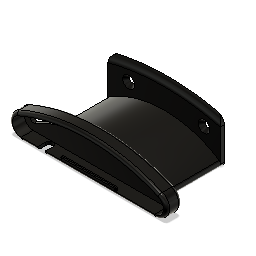
Logitech_g535_Wall_Mount (Autodesk Fusion 360 design; units mm, degrees)
Autodesk Fusion 360 part; units mm, degrees
note: some values were not read from the file. Set by a fixed rule: which face or edge a step refers to.
sketch "Sketch1" plane through (0, 0, 0) normal (0, 0, 1) x (1, 0, 0)
  line L0 (0, 0) -> (101.6, 0)
  line L1 (50.8, 0) -> (50.8, 17.4625)
  arc A0 (101.6, 0) -> (0, 0) centre (50.8, -65.1597) ccw
  dimension "d1" = 101.6
  dimension "d2" = 17.4625
  constraint coincident L0.start A0.end
  constraint horizontal L0
  constraint midpoint L0 L1.start
  constraint perpendicular L0 L1
  constraint coincident L1.end A0
  measures "d1" distance of L0.start L0.end
  measures "d2" distance of L1.start L1.end
extrude "Extrude1" add sketch "Sketch1" along normal blind 50.8 makes body 1
sketch "Sketch2" plane through (0, 0, 50.8) normal (0, 0, 1) x (1, 0, 0)
  arc A0 (101.6, 0) -> (0, 0) centre (50.8, -65.1597) ccw
  line L0 (0, 0) -> (101.6, 0)
  line L1 (0, 0) -> (101.6, 0)
  constraint coincident A0.end L0.start
  constraint coincident A0.start L0.end
copy_body "CopyPasteBodies1" bodies 1 makes body 2
move_body "Move1" bodies 2 to x (1, 0, 0) y (0, 1, 0) z (0, 0, 1) at (0, 40.64, 0)
scale "Scale1" factor 1.453488 about (0, 40.64, 0) bodies 2
sketch "Sketch3" plane through (0, 0, 0) normal (0, 0, -1) x (-1, 0, 0)
  arc A0 (0, 0) -> (-101.6, 0) centre (-50.8, -65.1597) ccw
  line L0 (-101.6, 0) -> (0, 0)
scale "Scale2" factor 1.5 about (0, 40.64, 0) bodies 2
sketch "Sketch4" plane through (0, 0, 0) normal (0, 0, -1) x (-1, 0, 0)
  arc A0 (0, 40.64) -> (-221.5116, 40.64) centre (-110.7558, -101.4232) ccw
  line L0 (-221.5116, 40.64) -> (0, 40.64)
fillet "Fillet1" radius 2.54 2 edges at (0, 0, 25.4) (101.6, 0, 25.4) on bodies 1
copy_body "Body->Comp1" bodies 1 removing the originals makes body 3 in component "Component"
copy_body "Body->Comp2" bodies 2 removing the originals makes body 4 in component "Component'"
scale "Scale1'" factor 0.8 about (221.5116, 40.64, 0) bodies 4 in component "Component'"
fillet "Fillet1'" radius 9.652 2 edges at (44.3023, 40.64, 44.3023) (221.5116, 40.64, 44.3023) on bodies 4 in component "Component'"
extrude "Extrude1'" cut 1 faces at (132.907, 50.7926, 88.6047) along direction (0, 0, -1) blind 76.2 on bodies 4 bodies 4 in component "Component'"
fillet "Fillet2" radius 2.54 8 edges at (132.907, 40.64, 0) (195.9758, 48.3263, 0) (132.907, 71.0978, 0) (69.8382, 48.3263, 0) (132.907, 40.64, 12.4047) (69.8382, 48.3263, 12.4047) (132.907, 71.0978, 12.4047) (195.9758, 48.3263, 12.4047) on bodies 4 in component "Component'"
extrude "Extrude2" cut 1 faces at (132.907, 51.6393, 12.4047) along direction (0, 0, -1) blind 9.652 on bodies 4 bodies 4 in component "Component'"
sketch "Sketch5" plane through (0, 0, 49.0633) normal (0, 0, -1) x (-1, 0, 0)
  line L0 (-104.4191, 2.54) -> (2.8191, 2.54)
  arc A0 (2.8191, 2.54) -> (5.6552, 16.174) centre (2.8191, 9.652) ccw
  arc A1 (5.6552, 16.174) -> (-107.2552, 16.174) centre (-50.8, -113.6506) ccw
  arc A2 (-107.2552, 16.174) -> (-104.4191, 2.54) centre (-104.4191, 9.652) ccw
  arc A3 (1.9271, 8.0079) -> (-103.5271, 8.0079) centre (-50.8, -89.1764) ccw
  arc A4 (1.9271, 8.0079) -> (3.7111, 11.2961) centre (2.8191, 9.652) ccw
  arc A5 (3.7111, 11.2961) -> (-105.3111, 11.2961) centre (-50.8, -89.1764) ccw
  arc A6 (-105.3111, 11.2961) -> (-103.5271, 8.0079) centre (-104.4191, 9.652) ccw
  arc A7 (2.8191, 9.652) -> (-104.4191, 9.652) centre (-50.8, -89.1764) ccw construction
  constraint tangent A3 A4
  constraint tangent A4 A5
  constraint tangent A5 A6
  constraint tangent A3 A6
  constraint coincident A2.centre A6.centre
  constraint coincident A0.centre A4.centre
extrude "Extrude3" cut sketch "Sketch5" against normal blind 23.114 contours A3 A4 A5 A6 sketch seen with x (1, 0, 0) y (0, 1, 0) z (0, 0, 1) at (82.107, 40.64, -49.0633) bodies 4 in component "Component'"
sketch "Sketch6" plane through (0, 0, 0) normal (0, 0, -1) x (-1, 0, 0)
  arc A0 (-94.9342, 4.6873) -> (-93.5774, 0) centre (-93.5774, 2.54) ccw
  line L0 (-93.5774, 0) -> (-8.0226, 0)
  arc A1 (-8.0226, 0) -> (-6.6658, 4.6873) centre (-8.0226, 2.54) ccw
  arc A2 (-6.6658, 4.6873) -> (-94.9342, 4.6873) centre (-50.8, -65.1597) ccw
  line L1 (-93.5774, 0) -> (-8.0226, 0)
  line L2 (-8.0226, 0) -> (-8.0226, 39.4194)
  line L3 (-8.0226, 39.4194) -> (-93.5774, 39.4194)
  line L4 (-93.5774, 39.4194) -> (-93.5774, 0)
  constraint horizontal L1
  constraint vertical L2
  constraint horizontal L3
  constraint vertical L4
  constraint coincident A0.end L0.start
extrude "Extrude1''" add sketch "Sketch6" along normal blind 3.048 contours L0 A2 L1 L2 L4 | A2 L2 L3 L4 bodies 3 in component "Component"
extrude "Extrude2'" add 1 faces at (93.5774, 14.9819, -2.032) along direction (1, 0, 0) blind 2.54 on bodies 3 bodies 3 in component "Component"
extrude "Extrude3'" add 1 faces at (8.0226, 14.9819, -2.032) along direction (-1, 0, 0) blind 2.54 on bodies 3 bodies 3 in component "Component"
extrude "Extrude4" cut 1 faces at (5.9816, 0.499, 0) along direction (0, 0, -1) blind 9.652 on bodies 3 bodies 3 in component "Component"
extrude "Extrude5" cut 1 faces at (95.6184, 0.499, 0) along direction (0, 0, -1) blind 14.986 on bodies 3 bodies 3 in component "Component"
sketch "Sketch7" plane through (0, 0, 0) normal (0, 0, 1) x (1, 0, 0)
  arc A0 (94.9342, 4.6873) -> (6.6658, 4.6873) centre (50.8, -65.1597) ccw
  arc A1 (96.1174, 2.54) -> (94.9342, 4.6873) centre (93.5774, 2.54) ccw
  line L0 (96.1174, 2.54) -> (96.1174, 39.4194)
  line L1 (96.1174, 39.4194) -> (5.4826, 39.4194)
  line L2 (5.4826, 39.4194) -> (5.4826, 2.54)
  arc A2 (6.6658, 4.6873) -> (5.4826, 2.54) centre (8.0226, 2.54) ccw
  line L3 (96.1174, 33.7875) -> (5.4826, 33.7875)
  arc A3 (96.1174, 33.7875) -> (5.4826, 33.7875) centre (50.8, -145.722) ccw
  constraint coincident L0 L3.start
  constraint coincident L2 L3.end
  constraint perpendicular L2 L3
  constraint tangent L1 A3
extrude "Extrude6" cut sketch "Sketch7" against normal blind 21.082 contours L0 L1 A3 | L1 L2 A3 bodies 3 in component "Component"
fillet "Fillet1''" radius 6.731 3 edges at (96.1174, 33.7875, -1.524) (5.4826, 33.7875, -1.524) (50.8, 39.4194, 0) on bodies 3 in component "Component"
sketch "Sketch8" plane through (0, 0, 0) normal (0, 0, 1) x (1, 0, 0)
  arc A0 (96.1174, 27.9709) -> (5.4826, 27.9709) centre (50.8, -145.722) ccw
  line L0 (5.4826, 27.9709) -> (5.4826, 2.54)
  arc A1 (6.6658, 4.6873) -> (5.4826, 2.54) centre (8.0226, 2.54) ccw
  arc A2 (94.9342, 4.6873) -> (6.6658, 4.6873) centre (50.8, -65.1597) ccw
  arc A3 (96.1174, 2.54) -> (94.9342, 4.6873) centre (93.5774, 2.54) ccw
  line L1 (96.1174, 2.54) -> (96.1174, 27.9709)
  line L2 (50.8, 17.4625) -> (96.1174, 17.4625)
  line L3 (96.1174, 27.9709) -> (96.1174, 17.4625)
  line L4 (96.1174, 22.7167) -> (5.4826, 22.7167)
  line L5 (50.8, 22.7167) -> (96.1174, 22.7167)
  line L6 (50.8, 22.7167) -> (5.4826, 22.7167)
  constraint midpoint A2 L2.start
  constraint coincident L1 L2.end
  constraint tangent A2 L2
  constraint perpendicular L1 L2
  constraint coincident A0.start L1.end
  constraint midpoint L3 L4.start
  constraint coincident L0 L4.end
  constraint perpendicular L0 L4
  constraint midpoint L4 L5.start
hole "Hole1" at (22.0996, 22.7287, 0) direction (0, 0, -1) diameter 4.064 depth 25.4 tip angle 180 countersink diameter 9.525 countersink angle 82 bodies 3 in component "Component"
hole "Hole2" at (82.7054, 22.1317, 0) direction (0, 0, -1) diameter 4.064 depth 25.4 tip angle 180 countersink diameter 9.525 countersink angle 82 bodies 3 in component "Component"
sketch "Sketch9" plane through (0, 2.54, 0) normal (0, 1, 0) x (-1, 0, 0)
  line L0 (2.8191, 61.468) -> (-104.4191, 61.468)
  line L1 (-104.4191, 61.468) -> (-104.4191, 51.816)
  line L2 (-104.4191, 51.816) -> (2.8191, 51.816)
  line L3 (2.8191, 51.816) -> (2.8191, 61.468)
  line L4 (-10.1941, 61.468) -> (-16.5441, 61.468)
  line L5 (-16.5441, 61.468) -> (-16.5441, 55.118)
  line L6 (-16.5441, 55.118) -> (-10.1941, 55.118)
  line L7 (-10.1941, 55.118) -> (-10.1941, 61.468)
  arc A0 (-16.5441, 55.118) -> (-10.1941, 55.118) centre (-13.3691, 55.118) ccw
  line L8 (-10.1941, 55.118) -> (-10.4907, 62.8376)
  line L9 (-10.1941, 55.118) -> (-2.4688, 55.118) construction
  line L10 (-16.5441, 55.118) -> (-16.2421, 62.9814)
  line L11 (-16.5441, 55.118) -> (-24.4133, 55.118) construction
  dimension "d48" = 6.35
  dimension "d49" = 6.35
  dimension "d50" = 92.2
  dimension "d51" = 92.2
  constraint horizontal L4
  constraint vertical L5
  constraint horizontal L6
  constraint vertical L7
  constraint coincident L0 L4.start
  constraint tangent L7 A0
  constraint horizontal L9
  constraint horizontal L11
  measures "d48" distance of L4.start L4.end
  measures "d49" distance of L4.start L6.end
  measures "d50" angle of L8 L9
  measures "d51" angle of L10 L11
extrude "Extrude4'" cut sketch "Sketch9" against normal blind 3.048 contours L0 L4 L6 L8 L10 | L6 A0 sketch seen with x (1, 0, 0) y (0, 1, 0) z (0, 0, 1) at (82.107, 40.64, -49.0633) bodies 4 in component "Component'"
sketch "Sketch10" plane through (0, 0, 51.816) normal (0, 0, 1) x (1, 0, 0)
  arc A0 (105.3111, 11.2961) -> (-3.7111, 11.2961) centre (50.8, -89.1764) ccw
  arc A1 (103.5271, 8.0079) -> (105.3111, 11.2961) centre (104.4191, 9.652) ccw
  arc A2 (103.5271, 8.0079) -> (-1.9271, 8.0079) centre (50.8, -89.1764) ccw
  arc A3 (-3.7111, 11.2961) -> (-1.9271, 8.0079) centre (-2.8191, 9.652) ccw
  line L0 (-2.8191, 2.54) -> (104.4191, 2.54)
  arc A4 (104.4191, 2.54) -> (107.2552, 16.174) centre (104.4191, 9.652) ccw
  arc A5 (107.2552, 16.174) -> (-5.6552, 16.174) centre (50.8, -113.6506) ccw
  arc A6 (-5.6552, 16.174) -> (-2.8191, 2.54) centre (-2.8191, 9.652) ccw
sketch "Sketch11" plane through (0, 2.54, 0) normal (0, 1, 0) x (-1, 0, 0)
  line L0 (-10.4381, 61.468) -> (-10.1941, 55.118)
  arc A0 (-16.5441, 55.118) -> (-10.1941, 55.118) centre (-13.3691, 55.118) ccw
  line L1 (-16.5441, 55.118) -> (-16.3002, 61.468)
  line L2 (-16.3002, 61.468) -> (-104.4191, 61.468)
  line L3 (-104.4191, 61.468) -> (-104.4191, 51.816)
  line L4 (-104.4191, 51.816) -> (2.8191, 51.816)
  line L5 (2.8191, 51.816) -> (2.8191, 61.468)
  line L6 (2.8191, 61.468) -> (-10.4381, 61.468)
  line L7 (2.8191, 56.642) -> (-104.4191, 56.642)
  line L8 (-50.8, 56.642) -> (-50.8, 61.468)
  line L9 (-50.8, 61.468) -> (-28.575, 61.468)
  line L10 (-28.575, 61.468) -> (-73.025, 61.468)
  line L11 (-73.025, 61.468) -> (-73.025, 59.8805)
  line L12 (-73.025, 59.8805) -> (-28.575, 59.8805)
  line L13 (-28.575, 59.8805) -> (-28.575, 61.468)
  dimension "d54" = 22.225
  dimension "d55" = 44.45
  dimension "d56" = 1.5875
  constraint midpoint L5 L7.start
  constraint midpoint L3 L7.end
  constraint midpoint L7 L8.start
  constraint coincident L2 L8.end
  constraint perpendicular L2 L8
  constraint perpendicular L8 L9
  constraint horizontal L10
  constraint vertical L11
  constraint horizontal L12
  constraint vertical L13
  measures "d54" distance of L8.end L9.end
  measures "d55" distance of L9.end L10.end
  measures "d56" distance of L9.end L12.end
extrude "Extrude5'" add sketch "Sketch11" along normal blind 2.54 contours L2 L8 L9 L10 L12 L13 | L2 L8 L10 L11 L12 sketch seen with x (1, 0, 0) y (0, 1, 0) z (0, 0, 1) at (82.107, 40.64, -49.0633) bodies 4 in component "Component'"
fillet "Fillet3" radius 0.635 5 edges at (132.907, 45.72, 12.4047) (110.682, 45.72, 11.6109) (110.682, 44.45, 12.4047) (155.132, 45.72, 11.6109) (155.132, 44.45, 12.4047) on bodies 4 in component "Component'"
component "Component" placed x (1, 0, 0) y (0, 1, 0) z (0, 0, 1) at (0, 0, 0)
component "Component'" placed x (1, 0, 0) y (0, 1, 0) z (0, 0, 1) at (-82.107, -40.64, 49.0633)
equation "d2 = ( 11 / 16 ) * 1 in"
equation "d5 = 1 / 0.688"
equation "d41 = ( 3 / 8 ) * 1 in"
equation "d54 = ( 1.75 / 2 ) * 1 in"
equation "d56 = ( 1 / 16 ) * 1 in"
